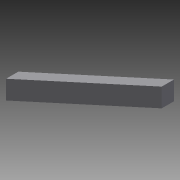
# Autodesk Inventor part: BallGuideLeft
Saved by Autodesk Inventor 2014 (Build 180170000, 170)
## iProperties
Created: 2016-02-06
Part Number: BallGuideLeft
Material: Generic
Document SubType Name: Modeling
Designer: choices
Density: 1 g/cm^3
Appearance: Default
Author: choices
Autodesk Inventor part; units mm, degrees
ref_plane "YZ Plane" through (0, 0, 0) normal (1, 0, 0) x (0, 1, 0)
ref_plane "XZ Plane" through (0, 0, 0) normal (0, 1, 0) x (-1, 0, 0)
ref_plane "XY Plane" through (0, 0, 0) normal (0, 0, 1) x (1, 0, 0)
sketch "Sketch1" plane through (0, 0, 0) normal (0, 1, 0) x (-1, 0, 0)
  line L0 (-102.9648, -88.0589) -> (68.4598, 55.7834)
  line L1 (-102.9648, -88.0589) -> (120.8142, -88.0589) construction
  line L2 (-102.9648, -88.0589) -> (-115.2099, -73.4658)
  line L3 (-115.2099, -73.4658) -> (68.4598, 80.6514)
  line L4 (68.4598, 80.6514) -> (68.4598, 55.7834)
  line L5 (-102.9648, -88.0589) -> (-102.9648, -63.1909)
  point P0 (0, 0)
  dimension "d0" = 40
  dimension "d1" = 171.4246
  dimension "d2" = 19.05
  constraints: 12 end point, 3 perpendicular, 1 equal length, 1 horizontal, 1 parallel, 1 point on line
  measures "d0" angle of L1 L0
  measures "d1" horizontal distance of L0.end L0.start
  measures "d2" distance of L0.start L2.end
extrude "Extrusion1" add sketch "Sketch1" along normal blind 38.1 contours L5 L3 L4 L0
body "Solid1"
